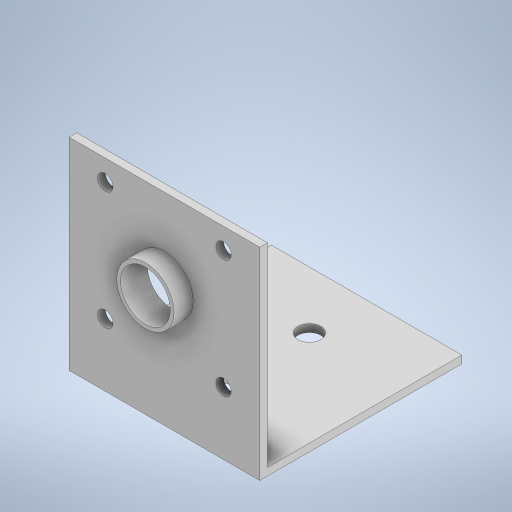
# Autodesk Inventor part: NEMA17-3030-m6-holder
Saved by Autodesk Inventor 2024 (Build 280153000, 153)
## iProperties
Created: 2025-12-08
Part Number: NEMA17-3030-m6-holder
Material: Generic
Document SubType Name: Modeling
Designer: schar
Density: 1 g/cm^3
Appearance: Default
Author: schar
Autodesk Inventor part; units mm, degrees
ref_plane "YZ Plane" through (0, 0, 0) normal (1, 0, 0) x (0, 1, 0)
ref_plane "XZ Plane" through (0, 0, 0) normal (0, 1, 0) x (-1, 0, 0)
ref_plane "XY Plane" through (0, 0, 0) normal (0, 0, 1) x (1, 0, 0)
sketch "Sketch1" plane through (0, 0, 0) normal (1, 0, 0) x (0, 1, 0)
  line L0 (0, 0) -> (51, 0)
  line L1 (51, 0) -> (51, 2)
  line L2 (51, 2) -> (0, 2)
  line L3 (-2, 0) -> (-2, -51)
  line L4 (-2, -51) -> (0, -51)
  line L5 (0, -51) -> (0, 0)
  line L6 (0, 0) -> (-2, 0)
  line L7 (-2, 0) -> (-2, 2)
  line L8 (-2, 2) -> (0, 2)
  line L9 (0, 2) -> (0, 0)
  dimension "d0" = 51
  dimension "d1" = 2
  dimension "d2" = 2
  dimension "d3" = 51
  constraints: 20 end point, 4 parallel, 2 horizontal, 2 perpendicular
  measures "d0" distance of L2.end L1.end
  measures "d1" distance of L1.end L0.end
  measures "d2" distance of L4.end L3.end
  measures "d3" distance of L3.end L3.start
extrude "Extrusion1" add sketch "Sketch1" along normal blind 50
sketch "Sketch2" plane through (0, 0, 0) normal (0, 0, -1) x (-1, 0, 0)
  line L0 (0, 51) -> (-50, 51) projected
  line L1 (-25, 51) -> (-25, 30)
  circle A0 centre (-25, 30) radius 6.5
  line L2 (-25, 51) -> (-9.5, 51)
  line L3 (-25, 30) -> (-9.5, 30)
  line L4 (-9.5, 30) -> (-9.5, 45.5)
  line L5 (-9.5, 30) -> (-9.5, 14.5)
  circle A1 centre (-9.5, 14.5) radius 2
  circle A2 centre (-9.5, 45.5) radius 2
  circle A3 centre (-40.5, 14.5) radius 2
  circle A4 centre (-40.5, 45.5) radius 2
  point P0 (0, 0)
  dimension "d6" = 21
  dimension "d7" = 13
  dimension "d8" = 15.5
  dimension "d9" = 15.5
  dimension "d10" = 15.5
  dimension "d11" = 4
  dimension "d12" = 4
  constraints: 10 end point, 5 centre point, 3 coincident, 2 symmetric about line, 2 vertical, 1 horizontal, 1 midpoint, 1 perpendicular, 1 point on line, 2 other
  measures "d6" distance of L1.start L1.end
  measures "d7" diameter of A0
  measures "d8" distance of L1.start L2.end
  measures "d9" distance of L3.end L4.end
  measures "d10" distance of L3.end L5.end
  measures "d11" diameter of A1
  measures "d12" diameter of A2
extrude "Extrusion2" cut sketch "Sketch2" against normal blind 50
sketch "Sketch3" plane through (0, 0, 0) normal (0, 1, 0) x (1, 0, 0)
  line L0 (0, 51) -> (50, 51) projected
  line L1 (25, 51) -> (25, 36)
  line L2 (25, 36) -> (25, 13)
  circle A0 centre (25, 13) radius 3
  circle A1 centre (25, 36) radius 3
  point P0 (0, 0)
  dimension "d15" = 15
  dimension "d16" = 23
  dimension "d17" = 6
  dimension "d18" = 6
  constraints: 4 end point, 2 centre point, 2 coincident, 1 midpoint, 1 point on line, 1 vertical
  measures "d15" distance of L1.start L1.end
  measures "d16" distance of L1.end L2.end
  measures "d17" diameter of A0
  measures "d18" diameter of A1
extrude "Extrusion3" cut sketch "Sketch3" against normal blind 50
sketch "Sketch4" plane through (0, -2, 2) normal (0, 0, 1) x (1, 0, 0)
  circle A0 centre (25, 32) radius 6.5 projected
  circle A1 centre (25, 32) radius 7.5
  circle A2 centre (25, 32) radius 6.5
  point P0 (0, 2)
  dimension "d21" = 15
  constraints: 2 centre point, 2 coincident, 1 concentric
  measures "d21" diameter of A1
extrude "Extrusion4" add sketch "Sketch4" along normal blind 5
body "Solid1"
